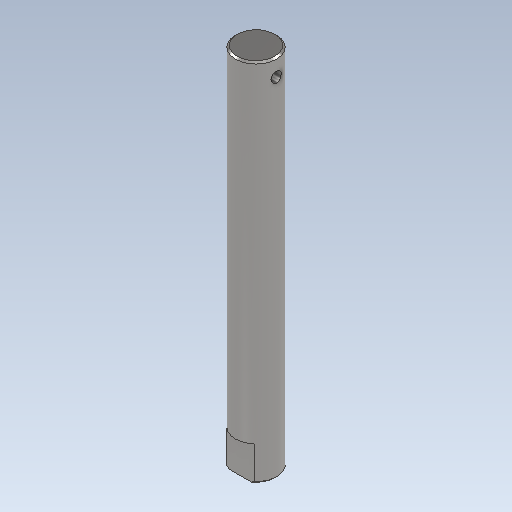
# Autodesk Inventor part: crankshaft
Saved by Autodesk Inventor 2020 (Build 240168000, 168)
## iProperties
Created: 2020-08-04
Part Number: crankshaft
Material: Stainless Steel
Document SubType Name: Modeling
Designer: benny
Density: 8 g/cm^3
Appearance: Semi-Polished
Author: benny
Autodesk Inventor part; units mm, degrees
ref_plane "YZ Plane" through (0, 0, 0) normal (1, 0, 0) x (0, 1, 0)
ref_plane "XZ Plane" through (0, 0, 0) normal (0, 1, 0) x (-1, 0, 0)
ref_plane "XY Plane" through (0, 0, 0) normal (0, 0, 1) x (1, 0, 0)
sketch "Sketch1" plane through (0, 0, 0) normal (0, 1, 0) x (-1, 0, 0)
  circle A0 centre (0, 0) radius 6
  dimension "d0" = 12
  constraints: 1 centre point, 1 coincident
  measures "d0" diameter of A0
extrude "Extrusion1" add sketch "Sketch1" along normal blind 105
sketch "Sketch2" plane through (0, 105, 0) normal (0, 1, 0) x (1, 0, 0)
  circle A0 centre (0, 0) radius 6
  dimension "d3" = 12
  constraints: 1 centre point, 1 coincident
  measures "d3" diameter of A0
extrude "Extrusion2" add sketch "Sketch2" along normal blind 0.5 draft -45
sketch "Sketch3" plane through (0, 0, 0) normal (0, -1, 0) x (1, 0, 0)
  circle A0 centre (0, 0) radius 6
  dimension "d6" = 12
  constraints: 1 centre point, 1 coincident
  measures "d6" diameter of A0
extrude "Extrusion3" add sketch "Sketch3" along normal blind 0.5 draft -45
sketch "Sketch4" plane through (0, -0.5, 0) normal (0, -1, 0) x (1, 0, 0)
  line L0 (-8.7277, 6) -> (8.7277, 6)
  line L1 (8.7277, 6) -> (8.7277, 4.5)
  line L2 (8.7277, 4.5) -> (-8.7277, 4.5)
  line L3 (-8.7277, 4.5) -> (-8.7277, 6)
  line L4 (-8.7277, 6) -> (8.7277, 4.5) construction
  line L5 (8.7277, 6) -> (-8.7277, 4.5) construction
  point P0 (0, 0)
  point P1 (0, 5.25)
  dimension "d9" = 1.5
  constraints: 12 end point, 2 midpoint, 2 parallel, 1 horizontal, 1 perpendicular
  measures "d9" distance of L0.end L1.end
extrude "Extrusion4" cut sketch "Sketch4" against normal blind 10
sketch "Sketch6" plane through (0, 0, 0) normal (1, 0, 0) x (0, 1, 0)
  circle A0 centre (100.5, 0) radius 1.5
  point P0 (0, 0)
  dimension "d15" = 3
  constraints: 1 centre point
  measures "d15" diameter of A0
extrude "Extrusion6" cut sketch "Sketch6" against normal mid plane 120
body "Solid1"
